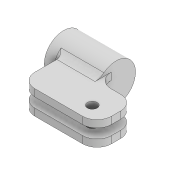
# Autodesk Inventor part: Hinge_5
Saved by Autodesk Inventor 2022 (Build 260153000, 153)
## iProperties
Created: 2022-07-08
Part Number: Hinge_5
Material: Generic
Document SubType Name: Modeling
Designer: dell
Density: 1 g/cm^3
Appearance: Default
Author: dell
Autodesk Inventor part; units mm, degrees
ref_plane "YZ Plane" through (0, 0, 0) normal (1, 0, 0) x (0, 1, 0)
ref_plane "XZ Plane" through (0, 0, 0) normal (0, 1, 0) x (-1, 0, 0)
ref_plane "XY Plane" through (0, 0, 0) normal (0, 0, 1) x (1, 0, 0)
sketch "Sketch1" plane through (0, 0, 0) normal (1, 0, 0) x (0, 1, 0)
  circle A0 centre (0, 0) radius 4.9
  circle A1 centre (0, 0) radius 6.1
  circle A2 centre (0, 0) radius 8.1
  dimension "d0" = 9.8
  dimension "d1" = 12.2
  dimension "d2" = 2
  constraints: 3 centre point, 2 coincident
  measures "d0" diameter of A0
  measures "d1" diameter of A1
  measures "d2" radial gap between concentric circles of A1 A2
extrude "Extrusion1" add sketch "Sketch1" along normal blind 20
sketch "Sketch2" plane through (20, 0, 0) normal (1, 0, 0) x (0, 0, -1)
  circle A0 centre (0, 0) radius 8.1 projected
  circle A1 centre (0, 0) radius 6.1 projected
extrude "Extrusion2" add sketch "Sketch2" along normal blind 2 contours A0 | A1
sketch "Sketch6" plane through (20, 0, 0) normal (-1, 0, 0) x (0, 0, 1)
  circle A0 centre (0, 0) radius 4.9 projected
  circle A1 centre (0, 0) radius 6.1 projected
sketch "Sketch11" plane through (22, 0, 0) normal (1, 0, 0) x (0, 0, -1)
  line L0 (-24, 5) -> (0, 5)
  line L1 (0, 5) -> (0, 2)
  line L2 (0, 2) -> (-24, 2)
  line L3 (-24, 2) -> (-24, 5)
  point P0 (0, 0)
  dimension "d57" = 2
  dimension "d58" = 3
  dimension "d60" = 24
  constraints: 8 end point, 2 parallel, 1 horizontal, 1 perpendicular, 1 point on line
  measures "d57" distance from line of point (0, 0) L2
  measures "d58" distance between parallel lines of L2 L0
  measures "d60" distance between parallel lines of L1 L3
extrude "Extrusion9" add sketch "Sketch11" along normal mid plane 32
sketch "Sketch12" plane through (22, 5, 6.3726) normal (0, 1, 0) x (1, 0, 0)
  circle A0 centre (8, -11.6274) radius 2.05
  line L0 (16, 6.3726) -> (16, -17.6274) projected
  line L1 (-16, -17.6274) -> (16, -17.6274) projected
  line L2 (16, -17.6274) -> (16, 6.3726) projected
  point P0 (-22, 6.3726)
  dimension "d63" = 4.1
  dimension "d64" = 8
  dimension "d65" = 6
  constraints: 1 centre point
  measures "d63" diameter of A0
  measures "d64" distance from line of L0 A0.centre
  measures "d65" distance from line of L1 A0.centre
extrude "Extrusion10" cut sketch "Sketch12" against normal blind 32
fillet "Fillet5" radius 6 3 edges at (6, 3.5, 24) (38, 3.5, 24) (14, 5, 6.3726)
fillet "Fillet6" radius 2 2 edges at (14, 2, 7.8492) (6, 4.386, 6.8098)
mirror "Mirror1" about plane through (0, 0, 0) normal (0, 1, 0) of "Extrusion9", "Extrusion10", "Fillet5", "Fillet6"
sketch "Sketch14" plane through (22, 0, 0) normal (1, 0, 0) x (0, 0, -1)
  line L0 (8.1, -8.1) -> (-8.1, -8.1)
  line L1 (-8.1, -8.1) -> (-8.1, 8.1)
  line L2 (-8.1, 8.1) -> (8.1, 8.1)
  line L3 (8.1, 8.1) -> (8.1, -8.1)
  line L4 (8.1, -8.1) -> (-8.1, 8.1) construction
  line L5 (-8.1, -8.1) -> (8.1, 8.1) construction
  point P0 (0, 0)
  dimension "d70" = 16.2
  dimension "d71" = 16.2
  constraints: 12 end point, 2 midpoint, 2 parallel, 1 horizontal, 1 perpendicular
  measures "d70" distance of L1.end L2.end
  measures "d71" distance of L0.end L1.end
extrude "Extrusion11" cut sketch "Sketch14" along normal blind 100
extrude "Extrusion12" cut sketch "Sketch6" along normal blind 100
fillet "Fillet7" radius 6 4 edges at (22, 3.5, 8.1) (22, -3.5, 8.1) (38, 3.5, 8.1) (38, -3.5, 8.1)
body "Solid1"
